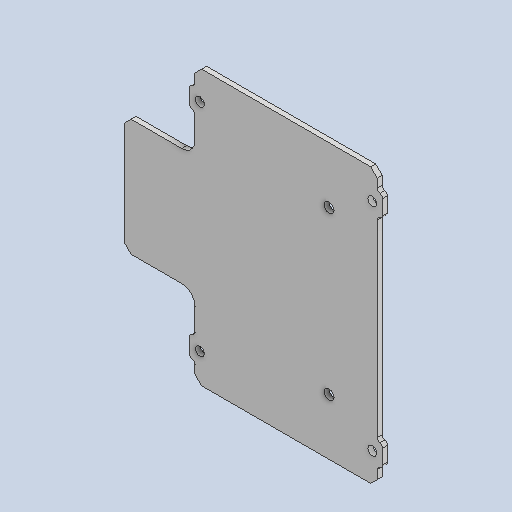
# Autodesk Inventor part: power_board
Saved by Autodesk Inventor 2025 (Build 290162000, 162)
## iProperties
Created: 2026-08-11
Part Number: power_board
Material: Типовые
Document SubType Name: Modeling
Designer: garin
Density: 1 g/cm^3
Appearance: По умолчанию
Author: garin
Autodesk Inventor part; units mm, degrees
ref_plane "YZ Plane" through (0, 0, 0) normal (1, 0, 0) x (0, 1, 0)
ref_plane "XZ Plane" through (0, 0, 0) normal (0, 1, 0) x (-1, 0, 0)
ref_plane "XY Plane" through (0, 0, 0) normal (0, 0, 1) x (1, 0, 0)
sketch "Эскиз1" plane through (0, 0, 0) normal (0, 0, 1) x (1, 0, 0)
  line L0 (-30, 41.5) -> (28, 41.5)
  line L1 (30, 39.5) -> (30, -39.5)
  line L2 (28, -41.5) -> (-30, -41.5)
  line L3 (-30, -41.5) -> (-30, 41.5)
  line L4 (-30, 41.5) -> (30, -41.5) construction
  line L5 (30, 41.5) -> (-30, -41.5) construction
  line L6 (-30, -41.5) -> (-42.5, -41.5)
  line L7 (-46.5, -37.5) -> (-46.5, 37.5)
  line L8 (-42.5, 41.5) -> (-30, 41.5)
  line L9 (-30, 41.5) -> (-30, -41.5)
  line L10 (-42.5, -41.5) -> (-46.5, -37.5)
  line L11 (-46.5, 37.5) -> (-42.5, 41.5)
  line L12 (28, 41.5) -> (30, 39.5)
  line L13 (28, -41.5) -> (30, -39.5)
  line L14 (0, 0) -> (-23.984, 0) construction
  line L15 (-23.984, 0) -> (-23.984, 15.7) construction
  line L16 (-23.984, 15.7) -> (0, 15.7) construction
  line L17 (0, 15.7) -> (0, 0) construction
  circle A0 centre (-23.984, 15.7) radius 1.6
  circle A1 centre (-23.984, -15.7) radius 1.6
  circle A2 centre (23.984, 15.7) radius 1.6
  circle A3 centre (23.984, -15.7) radius 1.6
  line L18 (-46.5, -41.5) -> (-25.168, -41.5)
  line L19 (-25.168, -41.5) -> (-25.168, -21.7)
  line L20 (-29.168, -17.7) -> (-46.5, -17.7)
  line L21 (-46.5, -17.7) -> (-46.5, -41.5)
  arc A4 (-25.168, -21.7) -> (-29.168, -17.7) centre (-29.168, -21.7) ccw
  line L22 (-25.168, 41.5) -> (-25.168, 21.7)
  line L23 (-29.168, 17.7) -> (-46.5, 17.7)
  arc A5 (-29.168, 17.7) -> (-25.168, 21.7) centre (-29.168, 21.7) ccw
  point P0 (-46.5, 41.5)
  point P1 (-25.168, -17.7)
  point P2 (-25.168, 41.5)
  point P3 (-46.5, -17.7)
  point P4 (-25.168, -41.5)
  dimension "d0" = 60
  dimension "d1" = 83
  dimension "d2" = 16.5
  dimension "d3" = 83
  dimension "d6" = 4
  dimension "d7" = 4
  dimension "d8" = 4
  dimension "d9" = 4
  dimension "d10" = 2
  dimension "d11" = 2
  dimension "d12" = 2
  dimension "d13" = 2
  dimension "d14" = 23.984
  dimension "d15" = 15.7
  dimension "d16" = 3.2
  dimension "d17" = 21.332
  dimension "d18" = 23.8
  dimension "d19" = 4
  constraints: 48 end point, 10 point on line, 8 parallel, 8 symmetric about line, 6 centre point, 4 horizontal, 4 perpendicular, 4 point on circle, 2 midpoint, 2 tangent, 1 coincident, 4 other
  measures "d0" distance of L4.end L2.end
  measures "d1" distance of L5.start L4.end
  measures "d2" distance of point (-46.5, 41.5) L8.end
  measures "d3" distance of L18.start point (-46.5, 41.5)
  measures "d6" distance of L6.end L18.start
  measures "d7" distance of L7.start L18.start
  measures "d8" distance of L7.end point (-46.5, 41.5)
  measures "d9" distance of L8.start point (-46.5, 41.5)
  measures "d10" distance of L0.end L5.start
  measures "d11" distance of L1.start L5.start
  measures "d12" distance of L2.start L4.end
  measures "d13" distance of L1.end L4.end
  measures "d14" distance of L15.end L16.end
  measures "d15" distance of L14.end L15.end
  measures "d16" diameter of A0
  measures "d17" distance of L20.end point (-25.168, -17.7)
  measures "d18" distance of point (-25.168, -17.7) L18.end
  measures "d19" radius of A4
extrude "Выдавливание1" add sketch "Эскиз1" along normal blind 1.5 contours L0 L12 L1 L13 L2 L19 A4 L20 L3 L23 A5 L22 | L3 L20 L7 L23 | A0 | A1 | A2 | A3
chamfer "Фаска1" distance 2 angle 45 4 edges at (-46.5, -17.7, 0.75) (-46.5, 17.7, 0.75) (-25.168, -41.5, 0.75) (-25.168, 41.5, 0.75)
sketch "Эскиз2" plane through (0, 0, 0) normal (0, 0, -1) x (-1, 0, 0)
  arc A0 (43.584, 17.7) -> (47.584, 21.7) centre (43.584, 21.7) ccw
  arc A1 (26.768, 34.9) -> (25.968, 35.8798) centre (25.768, 34.9) ccw
  line L0 (26.768, 34.9) -> (26.768, 30.4596)
  arc A2 (25.968, 29.4798) -> (26.768, 30.4596) centre (25.768, 30.4596) ccw
  arc A3 (25.968, 29.4798) -> (25.168, 28.5) centre (26.168, 28.5) ccw
  line L1 (25.168, 28.5) -> (25.168, 21.7)
  arc A4 (25.168, 21.7) -> (29.168, 17.7) centre (29.168, 21.7) ccw
  line L2 (29.168, 17.7) -> (43.584, 17.7)
  arc A5 (43.584, 17.7) -> (47.584, 21.7) centre (43.584, 21.7) ccw
  line L3 (47.584, 21.7) -> (47.584, 39.2)
  line L4 (47.584, 39.2) -> (25.168, 39.2)
  line L5 (25.168, 39.2) -> (25.168, 36.8596)
  arc A6 (25.168, 36.8596) -> (25.968, 35.8798) centre (26.168, 36.8596) ccw
  line L6 (52.084, -4) -> (58.0913, -4)
  line L7 (58.0913, -4) -> (58.0913, -38.5)
  line L8 (58.0913, -38.5) -> (69.3773, -38.5)
  line L9 (69.3773, -38.5) -> (69.3773, 32.5)
  line L10 (69.3773, 32.5) -> (58.0913, 32.5)
  line L11 (58.0913, 32.5) -> (58.0913, 24)
  line L12 (58.0913, 24) -> (52.084, 24)
  line L13 (52.084, 24) -> (52.084, 13.5)
  line L14 (52.084, 13.5) -> (34.584, 13.5)
  arc A7 (34.584, 13.5) -> (34.584, 1.5) centre (34.584, 7.5) ccw
  line L15 (34.584, 1.5) -> (47.084, 1.5)
  line L16 (47.084, 1.5) -> (47.084, -3.7639)
  spline S0 degree 3 poles (48.084, -6) (47.8036, -5.6035) (47.4716, -5.1246) (47.1717, -4.4032) (47.084, -4.0595) (47.084, -3.7639) knots 0 0 0 0 0.621631 0.621631 1 1 1 1
  line L17 (51.084, -6) -> (48.084, -6)
  spline S1 degree 3 poles (52.084, -3.7639) (52.084, -4.0595) (51.9963, -4.4032) (51.6964, -5.1246) (51.3644, -5.6035) (51.084, -6) knots 0 0 0 0 0.378369 0.378369 1 1 1 1
  line L18 (52.084, -3.7639) -> (52.084, -4)
  line L19 (74.484, -42.6) -> (-79.316, -42.6)
  line L20 (-79.316, -42.6) -> (-79.316, 42.6)
  line L21 (6.584, 42.6) -> (74.484, 42.6)
  line L22 (74.484, 42.6) -> (74.484, -42.6)
  circle A8 centre (23.684, -32.7) radius 1.6
  circle A9 centre (23.684, 32.7) radius 1.6
  line L23 (20.484, 41.2) -> (6.584, 41.2)
  line L24 (-25.316, 41.2) -> (-25.316, -41.2)
  line L25 (-25.316, -41.2) -> (20.484, -41.2)
  line L26 (20.484, -41.2) -> (20.484, 41.2)
  circle A10 centre (-28.516, -32.7) radius 1.6
  circle A11 centre (-28.516, 32.7) radius 1.6
  arc A12 (-31.6, 30.4596) -> (-30.8, 29.4798) centre (-30.6, 30.4596) ccw
  line L27 (-31.6, 30.4596) -> (-31.6, 34.9404)
  arc A13 (-30.8, 35.9202) -> (-31.6, 34.9404) centre (-30.6, 34.9404) ccw
  arc A14 (-30.8, 35.9202) -> (-30, 36.9) centre (-31, 36.9) ccw
  line L28 (-30, 36.9) -> (-30, 39.2)
  line L29 (-30, 39.2) -> (-52.416, 39.2)
  line L30 (-52.416, 39.2) -> (-52.416, 21.7)
  arc A15 (-52.416, 21.7) -> (-48.416, 17.7) centre (-48.416, 21.7) ccw
  line L31 (-48.416, 17.7) -> (-34, 17.7)
  arc A16 (-34, 17.7) -> (-30, 21.7) centre (-34, 21.7) ccw
  line L32 (-30, 21.7) -> (-30, 28.5)
  arc A17 (-30, 28.5) -> (-30.8, 29.4798) centre (-31, 28.5) ccw
  arc A18 (-31.6, -34.9) -> (-30.8, -35.8798) centre (-30.6, -34.9) ccw
  line L33 (-31.6, -34.9) -> (-31.6, -30.4596)
  arc A19 (-30.8, -29.4798) -> (-31.6, -30.4596) centre (-30.6, -30.4596) ccw
  arc A20 (-30.8, -29.4798) -> (-30, -28.5) centre (-31, -28.5) ccw
  line L34 (-30, -28.5) -> (-30, -21.7)
  arc A21 (-30, -21.7) -> (-34, -17.7) centre (-34, -21.7) ccw
  line L35 (-34, -17.7) -> (-48.416, -17.7)
  arc A22 (-48.416, -17.7) -> (-52.416, -21.7) centre (-48.416, -21.7) ccw
  line L36 (-52.416, -21.7) -> (-52.416, -39.2)
  line L37 (-52.416, -39.2) -> (-30, -39.2)
  line L38 (-30, -39.2) -> (-30, -36.8596)
  arc A23 (-30, -36.8596) -> (-30.8, -35.8798) centre (-31, -36.8596) ccw
  arc A24 (25.968, -35.9202) -> (26.768, -34.9404) centre (25.768, -34.9404) ccw
  arc A25 (25.968, -35.9202) -> (25.168, -36.9) centre (26.168, -36.9) ccw
  line L39 (25.168, -36.9) -> (25.168, -39.2)
  line L40 (25.168, -39.2) -> (47.584, -39.2)
  line L41 (47.584, -39.2) -> (47.584, -21.7)
  arc A26 (47.584, -21.7) -> (43.584, -17.7) centre (43.584, -21.7) ccw
  line L42 (43.584, -17.7) -> (29.168, -17.7)
  arc A27 (29.168, -17.7) -> (25.168, -21.7) centre (29.168, -21.7) ccw
  line L43 (25.168, -21.7) -> (25.168, -28.5)
  arc A28 (25.168, -28.5) -> (25.968, -29.4798) centre (26.168, -28.5) ccw
  arc A29 (26.768, -30.4596) -> (25.968, -29.4798) centre (25.768, -30.4596) ccw
  line L44 (26.768, -30.4596) -> (26.768, -34.9404)
  line L45 (25.168, -39.2) -> (25.168, 39.2)
  line L46 (25.168, -21.7) -> (25.168, -39.5)
  line L47 (-30, 39.2) -> (-30, -39.2)
  line L48 (-11.416, 42.6) -> (-11.416, 41.2)
  line L49 (-11.416, 41.2) -> (-25.316, 41.2)
  line L50 (6.584, 41.2) -> (6.584, 42.6)
  line L51 (-79.316, 42.6) -> (-11.416, 42.6)
  point P0 (0, 0)
  constraints: 4 end point, 2 collinear
extrude "Выдавливание2" add sketch "Эскиз2" against normal blind 1.5 contours L45 A9 A6 A1 L0 A2 A3 | L45 A9 | A8 L45 | A8 L45 A28 A29 L44 A24 A25 | L47 A10 | A10 L47 A23 A18 L33 A19 A20 | L47 A11 | A11 L47 A17 A12 L27 A13 A14 picked at (25.1894, 32.5653) picked at (25.1894, -32.8347) picked at (-30.0289, -32.5985) picked at (-30.0289, 32.8015)
sketch "Эскиз3" plane through (0, 0, 0) normal (0, 0, -1) x (-1, 0, 0)
  arc A0 (26.768, 34.9) -> (25.968, 35.8798) centre (25.768, 34.9) ccw
  line L0 (26.768, 34.9) -> (26.768, 30.4596)
  arc A1 (25.968, 29.4798) -> (26.768, 30.4596) centre (25.768, 30.4596) ccw
  arc A2 (25.968, 29.4798) -> (25.168, 28.5) centre (26.168, 28.5) ccw
  line L1 (25.168, 28.5) -> (25.168, 21.7)
  arc A3 (25.168, 21.7) -> (29.168, 17.7) centre (29.168, 21.7) ccw
  line L2 (29.168, 17.7) -> (43.584, 17.7)
  arc A4 (43.584, 17.7) -> (47.584, 21.7) centre (43.584, 21.7) ccw
  line L3 (47.584, 21.7) -> (47.584, 39.2)
  line L4 (47.584, 39.2) -> (25.168, 39.2)
  line L5 (25.168, 39.2) -> (25.168, 36.8596)
  arc A5 (25.168, 36.8596) -> (25.968, 35.8798) centre (26.168, 36.8596) ccw
  line L6 (52.084, -4) -> (58.0913, -4)
  line L7 (58.0913, -4) -> (58.0913, -38.5)
  line L8 (58.0913, -38.5) -> (69.3773, -38.5)
  line L9 (69.3773, -38.5) -> (69.3773, 32.5)
  line L10 (69.3773, 32.5) -> (58.0913, 32.5)
  line L11 (58.0913, 32.5) -> (58.0913, 24)
  line L12 (58.0913, 24) -> (52.084, 24)
  line L13 (52.084, 24) -> (52.084, 13.5)
  line L14 (52.084, 13.5) -> (34.584, 13.5)
  arc A6 (34.584, 13.5) -> (34.584, 1.5) centre (34.584, 7.5) ccw
  line L15 (34.584, 1.5) -> (47.084, 1.5)
  line L16 (47.084, 1.5) -> (47.084, -3.7639)
  spline S0 degree 3 poles (48.084, -6) (47.8036, -5.6035) (47.4716, -5.1246) (47.1717, -4.4032) (47.084, -4.0595) (47.084, -3.7639) knots 0 0 0 0 0.621631 0.621631 1 1 1 1
  line L17 (51.084, -6) -> (48.084, -6)
  spline S1 degree 3 poles (52.084, -3.7639) (52.084, -4.0595) (51.9963, -4.4032) (51.6964, -5.1246) (51.3644, -5.6035) (51.084, -6) knots 0 0 0 0 0.378369 0.378369 1 1 1 1
  line L18 (52.084, -3.7639) -> (52.084, -4)
  line L19 (74.484, -42.6) -> (-79.316, -42.6)
  line L20 (-79.316, -42.6) -> (-79.316, 42.6)
  line L21 (6.584, 42.6) -> (74.484, 42.6)
  line L22 (74.484, 42.6) -> (74.484, -42.6)
  circle A7 centre (23.684, -32.7) radius 1.6
  circle A8 centre (23.684, 32.7) radius 1.6
  line L23 (20.484, 41.2) -> (6.584, 41.2)
  line L24 (-25.316, 41.2) -> (-25.316, -41.2)
  line L25 (-25.316, -41.2) -> (20.484, -41.2)
  line L26 (20.484, -41.2) -> (20.484, 41.2)
  circle A9 centre (-28.516, -32.7) radius 1.6
  circle A10 centre (-28.516, 32.7) radius 1.6
  arc A11 (-31.6, 30.4596) -> (-30.8, 29.4798) centre (-30.6, 30.4596) ccw
  line L27 (-31.6, 30.4596) -> (-31.6, 34.9404)
  arc A12 (-30.8, 35.9202) -> (-31.6, 34.9404) centre (-30.6, 34.9404) ccw
  arc A13 (-30.8, 35.9202) -> (-30, 36.9) centre (-31, 36.9) ccw
  line L28 (-30, 36.9) -> (-30, 39.2)
  line L29 (-30, 39.2) -> (-52.416, 39.2)
  line L30 (-52.416, 39.2) -> (-52.416, 21.7)
  arc A14 (-52.416, 21.7) -> (-48.416, 17.7) centre (-48.416, 21.7) ccw
  line L31 (-48.416, 17.7) -> (-34, 17.7)
  arc A15 (-34, 17.7) -> (-30, 21.7) centre (-34, 21.7) ccw
  line L32 (-30, 21.7) -> (-30, 28.5)
  arc A16 (-30, 28.5) -> (-30.8, 29.4798) centre (-31, 28.5) ccw
  arc A17 (-31.6, -34.9) -> (-30.8, -35.8798) centre (-30.6, -34.9) ccw
  line L33 (-31.6, -34.9) -> (-31.6, -30.4596)
  arc A18 (-30.8, -29.4798) -> (-31.6, -30.4596) centre (-30.6, -30.4596) ccw
  arc A19 (-30.8, -29.4798) -> (-30, -28.5) centre (-31, -28.5) ccw
  line L34 (-30, -28.5) -> (-30, -21.7)
  arc A20 (-30, -21.7) -> (-34, -17.7) centre (-34, -21.7) ccw
  line L35 (-34, -17.7) -> (-48.416, -17.7)
  arc A21 (-48.416, -17.7) -> (-52.416, -21.7) centre (-48.416, -21.7) ccw
  line L36 (-52.416, -21.7) -> (-52.416, -39.2)
  line L37 (-52.416, -39.2) -> (-30, -39.2)
  line L38 (-30, -39.2) -> (-30, -36.8596)
  arc A22 (-30, -36.8596) -> (-30.8, -35.8798) centre (-31, -36.8596) ccw
  arc A23 (25.968, -35.9202) -> (26.768, -34.9404) centre (25.768, -34.9404) ccw
  arc A24 (25.968, -35.9202) -> (25.168, -36.9) centre (26.168, -36.9) ccw
  line L39 (25.168, -36.9) -> (25.168, -39.2)
  line L40 (25.168, -39.2) -> (47.584, -39.2)
  line L41 (47.584, -39.2) -> (47.584, -21.7)
  arc A25 (47.584, -21.7) -> (43.584, -17.7) centre (43.584, -21.7) ccw
  line L42 (43.584, -17.7) -> (29.168, -17.7)
  arc A26 (29.168, -17.7) -> (25.168, -21.7) centre (29.168, -21.7) ccw
  line L43 (25.168, -21.7) -> (25.168, -28.5)
  arc A27 (25.168, -28.5) -> (25.968, -29.4798) centre (26.168, -28.5) ccw
  arc A28 (26.768, -30.4596) -> (25.968, -29.4798) centre (25.768, -30.4596) ccw
  line L44 (26.768, -30.4596) -> (26.768, -34.9404)
  line L45 (25.168, -39.5) -> (23.168, -41.5)
  line L46 (23.168, -41.5) -> (25.168, -41.5) construction
  line L47 (25.168, -41.5) -> (25.168, -39.5) construction
  line L48 (25.168, -39.5) -> (23.168, -39.5) construction
  line L49 (23.168, -39.5) -> (23.168, -41.5) construction
  line L50 (25.168, -41.5) -> (-15.416, -41.5) construction
  line L51 (-15.416, -41.5) -> (-15.416, -24.5) construction
  line L52 (-15.416, -24.5) -> (25.168, -24.5) construction
  line L53 (25.168, -24.5) -> (25.168, -41.5) construction
  circle A29 centre (-15.416, -24.5) radius 1.5
  line L54 (-25.316, 0) -> (20.484, 0) construction
  circle A30 centre (-15.416, 24.5) radius 1.5
  circle A31 centre (23.684, -32.7) radius 1.35
  circle A32 centre (-28.516, -32.7) radius 1.35
  circle A33 centre (-28.516, 32.7) radius 1.35
  circle A34 centre (23.684, 32.7) radius 1.35
  line L55 (-11.416, 42.6) -> (-11.416, 41.2)
  line L56 (-11.416, 41.2) -> (-25.316, 41.2)
  line L57 (6.584, 41.2) -> (6.584, 42.6)
  line L58 (-79.316, 42.6) -> (-11.416, 42.6)
  point P0 (0, 0)
  dimension "d25" = 40.584
  dimension "d26" = 17
  dimension "d27" = 3
  dimension "d28" = 2.7
  dimension "d29" = 2.7
  dimension "d30" = 2.7
  dimension "d31" = 2.7
  constraints: 18 end point, 6 centre point, 5 coincident, 4 parallel, 2 horizontal, 2 midpoint, 2 perpendicular, 1 symmetric about line, 1 other
  measures "d25" distance of L51.end L52.end
  measures "d26" distance of L50.end L51.end
  measures "d27" diameter of A29
  measures "d28" diameter of A31
  measures "d29" diameter of A32
  measures "d30" diameter of A33
  measures "d31" diameter of A34
extrude "Выдавливание3" cut sketch "Эскиз3" against normal blind 1.5 contours A29 | A30 | A31 | A32 | A33 | A34
equation "\"d7\" = d6"
equation "\"d9\" = d8"
equation "\"d11\" = d10"
